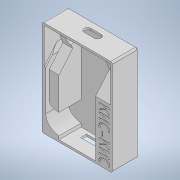
# Autodesk Inventor part: Корпус
Saved by Autodesk Inventor 2021.2 (Build 252289000, 289)
## iProperties
Created: 2023-10-18
Part Number: Корпус
Material: Типовые
Document SubType Name: Modeling
Designer: DELL
Density: 1 g/cm^3
Appearance: По умолчанию
Author: DELL
Autodesk Inventor part; units mm, degrees
ref_plane "YZ Plane" through (0, 0, 0) normal (1, 0, 0) x (0, 1, 0)
ref_plane "XZ Plane" through (0, 0, 0) normal (0, 1, 0) x (-1, 0, 0)
ref_plane "XY Plane" through (0, 0, 0) normal (0, 0, 1) x (1, 0, 0)
sketch "Эскиз1" plane through (0, 0, 0) normal (0, 0, 1) x (1, 0, 0)
  line L0 (10.25, -26.5) -> (-10.25, -26.5) construction
  line L1 (-10.25, -26.5) -> (-10.25, 26.5) construction
  line L2 (-10.25, 26.5) -> (10.25, 26.5) construction
  line L3 (10.25, 26.5) -> (10.25, -26.5) construction
  line L4 (10.25, -26.5) -> (-10.25, 26.5) construction
  line L5 (-10.25, -26.5) -> (10.25, 26.5) construction
  line L6 (19, 14.5) -> (-19, 14.5) construction
  line L7 (-19, 14.5) -> (-19, 26.5) construction
  line L8 (-19, 26.5) -> (19, 26.5) construction
  line L9 (19, 26.5) -> (19, 14.5) construction
  line L10 (19, 14.5) -> (-19, 26.5) construction
  line L11 (-19, 14.5) -> (19, 26.5) construction
  line L12 (-19.5, 14) -> (-10.75, 14)
  line L13 (-10.75, 14) -> (-10.75, -27)
  line L14 (-10.75, -27) -> (10.75, -27)
  line L15 (10.75, -27) -> (10.75, 14)
  line L16 (10.75, 14) -> (19.5, 14)
  line L17 (19.5, 14) -> (19.5, 27)
  line L18 (19.5, 27) -> (-19.5, 27)
  line L19 (-19.5, 27) -> (-19.5, 14)
  line L20 (0, 26.5) -> (0, -26.5) construction
  line L21 (20.7, -28.2) -> (-20.7, -28.2)
  line L22 (-20.7, -28.2) -> (-20.7, 28.2)
  line L23 (-20.7, 28.2) -> (20.7, 28.2)
  line L24 (20.7, 28.2) -> (20.7, -28.2)
  line L25 (20.7, -28.2) -> (-20.7, 28.2) construction
  line L26 (-20.7, -28.2) -> (20.7, 28.2) construction
  line L27 (-10.75, 14) -> (-10.75, 27)
  line L28 (10.75, 14) -> (10.75, 27)
  point P0 (0, 0)
  point P1 (0, 20.5)
  point P2 (0, 20.5)
  point P3 (0, 0)
  point P4 (0, 0)
  dimension "d0" = 20.5
  dimension "d1" = 53
  dimension "d2" = 38
  dimension "d3" = 12
  dimension "d4" = 0
  dimension "d5" = 0.5
  dimension "d8" = 0.5
  dimension "d9" = 0.5
  dimension "d10" = 0.5
  dimension "d11" = 0.5
  dimension "d13" = 1.2
  dimension "d14" = 1.2
  dimension "d15" = 1.2
  constraints: 60 end point, 11 midpoint, 10 perpendicular, 7 parallel, 5 horizontal, 3 point on line, 1 vertical alignment, 2 other
  measures "d0" distance of L1.end L2.end
  measures "d1" distance of L0.end L1.end
  measures "d2" distance of L7.end L8.end
  measures "d3" distance of L6.end L7.end
  measures "d4" distance between parallel lines of L2 L8
  measures "d5" distance between parallel lines of L19 L7
  measures "d8" distance between parallel lines of L18 L8
  measures "d9" distance between parallel lines of L6 L12
  measures "d10" distance between parallel lines of L1 L13
  measures "d11" distance between parallel lines of L0 L14
  measures "d13" distance between parallel lines of L23 L18
  measures "d14" distance between parallel lines of L22 L19
  measures "d15" distance between parallel lines of L14 L21
extrude "Выдавливание2" add sketch "Эскиз1" along normal blind 13 contours L19 L18 L27 L12 | L18 L17 L16 L28 | L21 L22 L23 L24
extrude "Выдавливание3" add sketch "Эскиз1" against normal blind 2 contours L19 L18 L27 L12 | L27 L18 L28 L15 L14 L13 | L18 L17 L16 L28 | L21 L22 L23 L24
fillet "Сопряжение1" radius 1 4 edges at (-20.7, 28.2, 5.5) (20.7, 28.2, 5.5) (-20.7, -28.2, 5.5) (20.7, -28.2, 5.5)
chamfer "Фаска1" distance 0.5 angle 45 8 edges at (20.7, 0, -2) (20.4071, -27.9071, -2) (0, -28.2, -2) (-20.4071, -27.9071, -2) (-20.7, 0, -2) (-20.4071, 27.9071, -2) (0, 28.2, -2) (20.4071, 27.9071, -2)
sketch "Эскиз7" plane through (0, 0, 0) normal (1, 0, 0) x (0, 1, 0)
  line L0 (27, 9.1171) -> (15.5358, 4.9445)
  line L1 (27, 9.1171) -> (27, 13)
  line L2 (27, 13) -> (5.9355, 13)
  line L3 (5.9355, 13) -> (15.5358, 4.9445)
  line L4 (27, 9.1171) -> (15.5358, 4.9445) construction
  line L5 (15.5358, 4.9445) -> (14.3045, 8.3274) construction
  line L6 (14.3045, 8.3274) -> (25.7687, 12.5) construction
  line L7 (25.7687, 12.5) -> (27, 9.1171) construction
  line L8 (27, 0) -> (-27, 0) construction
  line L9 (-27, 0) -> (-27, 13) construction
  line L10 (27, 13) -> (-27, 13) construction
  line L11 (27, 0) -> (27, 13) construction
  point P0 (0, 0)
  dimension "d57" = 120
  dimension "d58" = 12.2
  dimension "d59" = 3.6
  dimension "d64" = 0.5
  dimension "d65" = 20
  constraints: 16 end point, 3 equal length, 2 perpendicular, 1 vertical
  measures "d57" angle of L3 L0
  measures "d58" distance of L5.end L6.end
  measures "d59" distance of L6.end L0.start
  measures "d64" distance from line of L6.end L2
  measures "d65" angle of L0 L2
extrude "Выдавливание11" cut sketch "Эскиз7" against normal mid plane 39
sketch "Эскиз2" plane through (-19.7, 28.2, 13) normal (0, 1, 0) x (1, 0, 0)
  line L0 (22.7, 9) -> (16.7, 9) construction
  line L1 (22.7, 11) -> (16.7, 11)
  line L2 (16.7, 7) -> (22.7, 7)
  arc A0 (22.7, 7) -> (22.7, 11) centre (22.7, 9) ccw
  arc A1 (16.7, 11) -> (16.7, 7) centre (16.7, 9) ccw
  line L3 (8.95, 13) -> (8.95, 3.8829) construction
  line L4 (8.95, 13) -> (30.45, 13) construction
  line L5 (30.45, 13) -> (30.45, 3.8829) construction
  line L6 (30.45, 3.8829) -> (39.2, 3.8829) construction
  line L7 (39.2, 3.8829) -> (39.2, 0) construction
  line L8 (0.2, 0) -> (39.2, 0) construction
  line L9 (0.2, 0) -> (0.2, 3.8829) construction
  line L10 (0.2, 3.8829) -> (8.95, 3.8829) construction
  point P0 (19.7, 9)
  point P1 (19.7, 13)
  dimension "d26" = 10
  dimension "d27" = 4
  dimension "d66" = 2
  constraints: 8 end point, 4 point on circle, 4 tangent, 2 centre point, 2 midpoint, 1 parallel, 1 vertical alignment
  measures "d27" distance between parallel lines of L2 L1
  measures "d66" distance between parallel lines of L4 L1
extrude "Выдавливание4" cut sketch "Эскиз2" against normal up to next
sketch "Эскиз3" plane through (-19.7, 28.2, 13) normal (0, 0, 1) x (1, 0, 0)
  line L0 (38.5702, -23.6917) -> (38.5702, -54.9728) construction
  line L1 (38.5702, -54.9728) -> (32.2798, -54.9728) construction
  line L2 (32.2798, -54.9728) -> (32.2798, -23.6917) construction
  line L3 (32.2798, -23.6917) -> (38.5702, -23.6917) construction
  line L4 (16.7, 0) -> (22.7, 0) construction
  line L5 (0, -56.4) -> (39.4, -56.4) construction
  line L6 (39.2, -22.2645) -> (30.45, -22.2645) construction
  line L7 (40.4, -55.4) -> (40.4, -1) construction
  line L8 (30.45, -22.2645) -> (30.45, -55.2) construction
  line L9 (35.5731, -25.7166) -> (34.7773, -25.0517)
  line L10 (34.7773, -25.0517) -> (32.8531, -25.0517)
  spline S0 degree 2 poles (32.8531, -25.0517) (32.4702, -25.0517) (32.4702, -24.6689) knots 0 0 0 1 1 1
  spline S1 degree 2 poles (32.4702, -24.6689) (32.4702, -24.286) (32.8531, -24.286) knots 0 0 0 1 1 1
  line L11 (32.8531, -24.286) -> (38.1924, -24.286)
  spline S2 degree 2 poles (38.1924, -24.286) (38.5702, -24.286) (38.5702, -24.6689) knots 0 0 0 1 1 1
  spline S3 degree 2 poles (38.5702, -24.6689) (38.5702, -25.0517) (38.1924, -25.0517) knots 0 0 0 1 1 1
  line L12 (38.1924, -25.0517) -> (35.7847, -25.0517)
  line L13 (35.7847, -25.0517) -> (38.4443, -27.3486)
  spline S4 degree 2 poles (38.4443, -27.3486) (38.5702, -27.4595) (38.5702, -27.6358) knots 0 0 0 1 1 1
  spline S5 degree 2 poles (38.5702, -27.6358) (38.5702, -28.0186) (38.1924, -28.0186) knots 0 0 0 1 1 1
  spline S6 degree 2 poles (38.1924, -28.0186) (38.0464, -28.0186) (37.9053, -27.7919) knots 0 0 0 1 1 1
  line L14 (37.9053, -27.7919) -> (36.1121, -26.2405)
  line L15 (36.1121, -26.2405) -> (33.0394, -27.9632)
  spline S7 degree 2 poles (33.0394, -27.9632) (32.9488, -28.0186) (32.8531, -28.0186) knots 0 0 0 1 1 1
  spline S8 degree 2 poles (32.8531, -28.0186) (32.7019, -28.0186) (32.4702, -27.7818) (32.4702, -27.6358) knots 0 0 0 1 2 2 2
  spline S9 degree 2 poles (32.4702, -27.6358) (32.4702, -27.404) (32.7171, -27.2832) knots 0 0 0 1 1 1
  line L16 (32.7171, -27.2832) -> (35.5731, -25.7166)
  spline S10 degree 2 poles (38.5702, -32.3808) (38.5702, -32.7636) (38.1924, -32.7636) knots 0 0 0 1 1 1
  line L17 (38.1924, -32.7636) -> (32.8531, -32.7636)
  spline S11 degree 2 poles (32.8531, -32.7636) (32.4702, -32.7636) (32.4702, -32.3808) knots 0 0 0 1 1 1
  spline S12 degree 2 poles (32.4702, -32.3808) (32.4702, -31.9979) (32.8531, -31.9979) knots 0 0 0 1 1 1
  line L18 (32.8531, -31.9979) -> (36.7216, -31.9979)
  line L19 (36.7216, -31.9979) -> (33.1251, -29.8017)
  spline S13 degree 2 poles (33.1251, -29.8017) (32.8228, -29.8017) (32.7221, -29.7715) knots 0 0 0 1 1 1
  spline S14 degree 2 poles (32.7221, -29.7715) (32.4702, -29.706) (32.4702, -29.4189) knots 0 0 0 1 1 1
  spline S15 degree 2 poles (32.4702, -29.4189) (32.4702, -29.0361) (32.8531, -29.0361) knots 0 0 0 1 1 1
  line L20 (32.8531, -29.0361) -> (38.1924, -29.0361)
  spline S16 degree 2 poles (38.1924, -29.0361) (38.5702, -29.0361) (38.5702, -29.4189) knots 0 0 0 1 1 1
  spline S17 degree 2 poles (38.5702, -29.4189) (38.5702, -29.8017) (38.1924, -29.8017) knots 0 0 0 1 1 1
  line L21 (38.1924, -29.8017) -> (34.3239, -29.8017)
  line L22 (34.3239, -29.8017) -> (37.9204, -31.9979)
  spline S18 degree 2 poles (37.9204, -31.9979) (38.2227, -31.9979) (38.3184, -32.0231) knots 0 0 0 1 1 1
  spline S19 degree 2 poles (38.3184, -32.0231) (38.5702, -32.0886) (38.5702, -32.3808) knots 0 0 0 1 1 1
  spline S20 degree 2 poles (38.5702, -36.5415) (38.5702, -36.9243) (38.1924, -36.9243) knots 0 0 0 1 1 1
  spline S21 degree 2 poles (38.1924, -36.9243) (37.8096, -36.9243) (37.8096, -36.5415) knots 0 0 0 1 1 1
  line L23 (37.8096, -36.5415) -> (37.8096, -35.3577)
  spline S22 degree 2 poles (37.8096, -35.3577) (37.8096, -34.8943) (37.4117, -34.6626) knots 0 0 0 1 1 1
  spline S23 degree 2 poles (37.4117, -34.6626) (37.2253, -34.5518) (37.0037, -34.5518) knots 0 0 0 1 1 1
  line L24 (37.0037, -34.5518) -> (34.0418, -34.5518)
  spline S24 degree 2 poles (34.0418, -34.5518) (33.7043, -34.5518) (33.2308, -35.0253) (33.2308, -35.3577) knots 0 0 0 1 2 2 2
  line L25 (33.2308, -35.3577) -> (33.2308, -36.5415)
  spline S25 degree 2 poles (33.2308, -36.5415) (33.2308, -36.9243) (32.8531, -36.9243) knots 0 0 0 1 1 1
  spline S26 degree 2 poles (32.8531, -36.9243) (32.4702, -36.9243) (32.4702, -36.5415) knots 0 0 0 1 1 1
  line L26 (32.4702, -36.5415) -> (32.4702, -35.3577)
  spline S27 degree 2 poles (32.4702, -35.3577) (32.4702, -34.7029) (33.387, -33.7861) (34.0418, -33.7861) knots 0 0 0 1 2 2 2
  line L27 (34.0418, -33.7861) -> (37.0087, -33.7861)
  spline S28 degree 2 poles (37.0087, -33.7861) (37.6535, -33.7861) (38.5702, -34.7029) (38.5702, -35.3577) knots 0 0 0 1 2 2 2
  line L28 (38.5702, -35.3577) -> (38.5702, -36.5415)
  line L29 (33.9512, -40.6971) -> (33.9512, -38.3246)
  spline S29 degree 2 poles (33.9512, -38.3246) (33.9512, -37.9418) (34.334, -37.9418) knots 0 0 0 1 1 1
  spline S30 degree 2 poles (34.334, -37.9418) (34.7118, -37.9418) (34.7118, -38.3246) knots 0 0 0 1 1 1
  line L30 (34.7118, -38.3246) -> (34.7118, -40.6971)
  spline S31 degree 2 poles (34.7118, -40.6971) (34.7118, -41.0799) (34.334, -41.0799) knots 0 0 0 1 1 1
  spline S32 degree 2 poles (34.334, -41.0799) (33.9512, -41.0799) (33.9512, -40.6971) knots 0 0 0 1 1 1
  line L31 (35.5731, -43.528) -> (34.7773, -42.8631)
  line L32 (34.7773, -42.8631) -> (32.8531, -42.8631)
  spline S33 degree 2 poles (32.8531, -42.8631) (32.4702, -42.8631) (32.4702, -42.4803) knots 0 0 0 1 1 1
  spline S34 degree 2 poles (32.4702, -42.4803) (32.4702, -42.0974) (32.8531, -42.0974) knots 0 0 0 1 1 1
  line L33 (32.8531, -42.0974) -> (38.1924, -42.0974)
  spline S35 degree 2 poles (38.1924, -42.0974) (38.5702, -42.0974) (38.5702, -42.4803) knots 0 0 0 1 1 1
  spline S36 degree 2 poles (38.5702, -42.4803) (38.5702, -42.8631) (38.1924, -42.8631) knots 0 0 0 1 1 1
  line L34 (38.1924, -42.8631) -> (35.7847, -42.8631)
  line L35 (35.7847, -42.8631) -> (38.4443, -45.16)
  spline S37 degree 2 poles (38.4443, -45.16) (38.5702, -45.2709) (38.5702, -45.4472) knots 0 0 0 1 1 1
  spline S38 degree 2 poles (38.5702, -45.4472) (38.5702, -45.83) (38.1924, -45.83) knots 0 0 0 1 1 1
  spline S39 degree 2 poles (38.1924, -45.83) (38.0464, -45.83) (37.9053, -45.6033) knots 0 0 0 1 1 1
  line L36 (37.9053, -45.6033) -> (36.1121, -44.0519)
  line L37 (36.1121, -44.0519) -> (33.0394, -45.7746)
  spline S40 degree 2 poles (33.0394, -45.7746) (32.9488, -45.83) (32.8531, -45.83) knots 0 0 0 1 1 1
  spline S41 degree 2 poles (32.8531, -45.83) (32.7019, -45.83) (32.4702, -45.5932) (32.4702, -45.4472) knots 0 0 0 1 2 2 2
  spline S42 degree 2 poles (32.4702, -45.4472) (32.4702, -45.2154) (32.7171, -45.0946) knots 0 0 0 1 1 1
  line L38 (32.7171, -45.0946) -> (35.5731, -43.528)
  spline S43 degree 2 poles (38.5702, -50.1922) (38.5702, -50.575) (38.1924, -50.575) knots 0 0 0 1 1 1
  line L39 (38.1924, -50.575) -> (32.8531, -50.575)
  spline S44 degree 2 poles (32.8531, -50.575) (32.4702, -50.575) (32.4702, -50.1922) knots 0 0 0 1 1 1
  spline S45 degree 2 poles (32.4702, -50.1922) (32.4702, -49.8093) (32.8531, -49.8093) knots 0 0 0 1 1 1
  line L40 (32.8531, -49.8093) -> (36.7216, -49.8093)
  line L41 (36.7216, -49.8093) -> (33.1251, -47.6131)
  spline S46 degree 2 poles (33.1251, -47.6131) (32.8228, -47.6131) (32.7221, -47.5829) knots 0 0 0 1 1 1
  spline S47 degree 2 poles (32.7221, -47.5829) (32.4702, -47.5174) (32.4702, -47.2303) knots 0 0 0 1 1 1
  spline S48 degree 2 poles (32.4702, -47.2303) (32.4702, -46.8475) (32.8531, -46.8475) knots 0 0 0 1 1 1
  line L42 (32.8531, -46.8475) -> (38.1924, -46.8475)
  spline S49 degree 2 poles (38.1924, -46.8475) (38.5702, -46.8475) (38.5702, -47.2303) knots 0 0 0 1 1 1
  spline S50 degree 2 poles (38.5702, -47.2303) (38.5702, -47.6131) (38.1924, -47.6131) knots 0 0 0 1 1 1
  line L43 (38.1924, -47.6131) -> (34.3239, -47.6131)
  line L44 (34.3239, -47.6131) -> (37.9204, -49.8093)
  spline S51 degree 2 poles (37.9204, -49.8093) (38.2227, -49.8093) (38.3184, -49.8345) knots 0 0 0 1 1 1
  spline S52 degree 2 poles (38.3184, -49.8345) (38.5702, -49.9) (38.5702, -50.1922) knots 0 0 0 1 1 1
  spline S53 degree 2 poles (38.5702, -54.3528) (38.5702, -54.7357) (38.1924, -54.7357) knots 0 0 0 1 1 1
  spline S54 degree 2 poles (38.1924, -54.7357) (37.8096, -54.7357) (37.8096, -54.3528) knots 0 0 0 1 1 1
  line L45 (37.8096, -54.3528) -> (37.8096, -53.1691)
  spline S55 degree 2 poles (37.8096, -53.1691) (37.8096, -52.7057) (37.4117, -52.474) knots 0 0 0 1 1 1
  spline S56 degree 2 poles (37.4117, -52.474) (37.2253, -52.3632) (37.0037, -52.3632) knots 0 0 0 1 1 1
  line L46 (37.0037, -52.3632) -> (34.0418, -52.3632)
  spline S57 degree 2 poles (34.0418, -52.3632) (33.7043, -52.3632) (33.2308, -52.8367) (33.2308, -53.1691) knots 0 0 0 1 2 2 2
  line L47 (33.2308, -53.1691) -> (33.2308, -54.3528)
  spline S58 degree 2 poles (33.2308, -54.3528) (33.2308, -54.7357) (32.8531, -54.7357) knots 0 0 0 1 1 1
  spline S59 degree 2 poles (32.8531, -54.7357) (32.4702, -54.7357) (32.4702, -54.3528) knots 0 0 0 1 1 1
  line L48 (32.4702, -54.3528) -> (32.4702, -53.1691)
  spline S60 degree 2 poles (32.4702, -53.1691) (32.4702, -52.5143) (33.387, -51.5975) (34.0418, -51.5975) knots 0 0 0 1 2 2 2
  line L49 (34.0418, -51.5975) -> (37.0087, -51.5975)
  spline S61 degree 2 poles (37.0087, -51.5975) (37.6535, -51.5975) (38.5702, -52.5143) (38.5702, -53.1691) knots 0 0 0 1 2 2 2
  line L50 (38.5702, -53.1691) -> (38.5702, -54.3528)
  dimension "d67" = 31.2812
  dimension "d68" = 6.2905
  dimension "d69" = 1.4272
  dimension "d70" = 1.4272
  dimension "d71" = 1.8298
  dimension "d72" = 1.8298
  constraints: 2 other
  measures "d67" distance of L0.start L0.end
  measures "d68" distance of L0.end L1.end
  measures "d69" distance between parallel lines of L1 L5
  measures "d70" distance between parallel lines of L6 L3
  measures "d71" distance between parallel lines of L7 L0
  measures "d72" distance between parallel lines of L8 L2
emboss "Рельеф1" sketch "Эскиз3" operation cut depth 0.6 direction (0, 0, -1)
sketch "Эскиз4" plane through (-19.7, 28.2, 13) normal (0, 0, 1) x (1, 0, 0)
  line L0 (3.2, -1.2) -> (3.2, -14.2)
  line L1 (1.2, -17.8192) -> (1.2, -45.7113)
  line L2 (3.2, -37.8219) -> (3.2, -14.2)
  line L3 (8.95, -53.2) -> (3.0919, -52.2989) construction
  line L4 (3.0919, -52.2989) -> (1.2, -48.9154) construction
  line L5 (1.2, -48.9154) -> (1.2, -45.7113) construction
  spline S0 degree 3 poles (8.95, -53.2) (3.0919, -52.2989) (1.2, -48.9154) (1.2, -45.7113) knots 1 1 1 1 2 2 2 2
  line L6 (8.95, -41.2) -> (4.9393, -41.2) construction
  line L7 (4.9393, -41.2) -> (3.2, -39.7886) construction
  line L8 (3.2, -39.7886) -> (3.2, -37.8219) construction
  spline S1 degree 3 poles (8.95, -41.2) (4.9393, -41.2) (3.2, -39.7886) (3.2, -37.8219) knots 1 1 1 1 2 2 2 2
  line L9 (8.95, -53.2) -> (8.95, -41.2)
  line L10 (16.7, -1.2) -> (22.7, -1.2) construction
  line L11 (22.7, -1.2) -> (22.7, -1.2) construction
  line L12 (22.7, -1.2) -> (16.7, -1.2) construction
  line L13 (16.7, -1.2) -> (16.7, -1.2) construction
  line L14 (8.95, -1.2) -> (30.45, -1.2) construction
  line L15 (30.45, -1.2) -> (39.2, -1.2) construction
  line L16 (0.2, -1.2) -> (39.2, -1.2) construction
  line L17 (0.2, -1.2) -> (8.95, -1.2) construction
  line L18 (0.2, -22.2645) -> (0.2, -1.2) construction
  line L19 (0.2, -12.6642) -> (0.2, -22.2645) construction
  line L20 (0.2, -1.2) -> (0.2, -12.6642) construction
  line L21 (-1, -55.4) -> (-1, -1) construction
  line L22 (-1, -1) -> (-1, -55.4) construction
  line L23 (30.45, -55.2) -> (8.95, -55.2) construction
  line L24 (30.45, -55.2) -> (8.95, -55.2) construction
  line L25 (8.95, -12.6642) -> (8.95, -22.2645) construction
  line L26 (8.95, -55.2) -> (8.95, -22.2645) construction
  line L27 (8.95, -55.2) -> (8.95, -1.2) construction
  line L28 (8.95, -1.2) -> (8.95, -12.6642) construction
  line L29 (0.2, -1.2) -> (39.2, -1.2) construction
  line L30 (0.2, -1.2) -> (0.2, -13.2)
  line L31 (0.2, -12.6642) -> (0.2, -22.2645) construction
  line L32 (0.2, -1.2) -> (3.2, -1.2)
  line L33 (1.2, -17.8192) -> (1.2, -16.4245) construction
  line L34 (30.45, -1.2) -> (30.45, -55.2) construction
  line L35 (1.2, -16.4245) -> (0.2, -16.2472) construction
  line L36 (0.2, -16.2472) -> (0.2, -13.2) construction
  spline S2 degree 3 poles (1.2, -17.8192) (1.2, -16.4245) (0.2, -16.2472) (0.2, -13.2) knots 1 1 1 1 2 2 2 2
  point P0 (0.2, -1.2)
  dimension "d38" = 12
  dimension "d39" = 2
  dimension "d73" = 3
  dimension "d74" = 12
  constraints: 12 end point, 4 vertical, 2 horizontal, 2 point on line, 1 parallel, 1 perpendicular, 10 other
  measures "d38" distance of L6.start L3.start
  measures "d39" distance between parallel lines of L1 L2
  measures "d73" distance between parallel lines of L0 L18
  measures "d74" distance of L16.start L30.end
extrude "Выдавливание5" cut sketch "Эскиз4" against normal up to surface (13 mm away)
sketch "Эскиз6" plane through (-19.7, -28.2, 12) normal (0, -1, 0) x (1, 0, 0)
  line L0 (8.95, -12) -> (30.45, -12) construction
  line L1 (30.45, -12) -> (8.95, -12) construction
  line L2 (14.2, -6.5) -> (25.2, -6.5)
  line L3 (25.2, -6.5) -> (25.2, -10)
  line L4 (25.2, -10) -> (14.2, -10)
  line L5 (14.2, -10) -> (14.2, -6.5)
  line L6 (3.2, -12) -> (8.95, -12) projected
  line L7 (0.2, -12) -> (3.2, -12) projected
  line L8 (1.2, -12) -> (0.2, -12) projected
  line L9 (8.95, -12) -> (1.2, -12) projected
  point P0 (19.7, -12)
  point P1 (19.7, -10)
  dimension "d52" = 11
  dimension "d53" = 2
  dimension "d54" = 3.5
  constraints: 8 end point, 2 midpoint, 2 parallel, 1 horizontal, 1 perpendicular, 1 vertical alignment
  measures "d52" distance of L3.end L4.end
  measures "d53" distance between parallel lines of L0 L4
  measures "d54" distance of L4.end L2.start
extrude "Выдавливание10" cut sketch "Эскиз6" against normal up to next
sketch "Эскиз8" plane through (-16.5, 15.5358, 4.9445) normal (0, -0.3420201, 0.9396926) x (1, 0, 0)
  line L0 (0, 12.2) -> (0, 0) construction
  line L1 (0, 0) -> (5.75, 0) construction
  line L2 (5.75, 12.2) -> (5.75, 0) construction
  line L3 (0, 12.2) -> (5.75, 12.2) construction
  line L4 (5.75, 12.2) -> (5.75, 0) construction
  line L5 (5.75, 6.4) -> (3.6, 6.4)
  line L6 (3.6, 6.4) -> (3.6, 2.4)
  line L7 (3.6, 2.4) -> (5.75, 2.4)
  line L8 (5.75, 2.4) -> (5.75, 6.4)
  line L9 (-3, -2.1945) -> (-3, 9.0818) construction
  point P0 (16.5, -16.2899)
  dimension "d75" = 5.8
  dimension "d76" = 4
  dimension "d77" = 6.6
  constraints: 8 end point, 2 parallel, 1 horizontal, 1 perpendicular, 1 point on line
  measures "d75" distance between parallel lines of L3 L5
  measures "d76" distance of L5.end L6.end
  measures "d77" distance between parallel lines of L6 L9
extrude "Выдавливание12" cut sketch "Эскиз8" against normal blind 1.5
equation "\"d8\" = d5"
equation "\"d9\" = d5"
equation "\"d10\" = d5"
equation "\"d11\" = d5"
equation "\"d14\" = d13"
equation "\"d15\" = d13"
equation "\"d69\" = d70"
equation "\"d71\" = d72"
